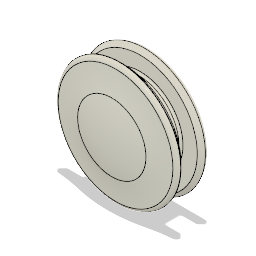
StepperBeltDisc v8 (Autodesk Fusion 360 design; units mm, degrees)
Autodesk Fusion 360 part; units mm, degrees
note: some values were not read from the file. Chosen so that the rebuilt part matches the saved one: which face or edge a step refers to; which pieces of a blend or face edit are solid. Set by a fixed rule: which sketch regions a step uses.
sketch "Sketch1" plane through (0, 0, 0) normal (0, 0, 1) x (1, 0, 0)
  circle A0 centre (0, 0) radius 15
  dimension "d1" = 30
  constraint coincident A0.centre origin
  measures "d1" diameter of A0
extrude "Extrude1" add sketch "Sketch1" along normal blind 8
sketch "Sketch2" plane through (0, 0, 0) normal (1, 0, 0) x (0, 0, -1)
  line L0 (0, 15) -> (0, -15)
  line L1 (-2, 15) -> (-2, 10)
  line L2 (-2, 10) -> (-6, 10)
  line L3 (-6, 10) -> (-6, 15)
  line L4 (-6, 15) -> (-2, 15)
  dimension "d4" = 5
  constraint parallel L0 L1
  constraint perpendicular L1 L2
  constraint perpendicular L2 L3
  constraint perpendicular L1 L4
  measures "d4" distance of L1.start L1.end
revolve "Revolve1" cut sketch "Sketch2" angle 360 about axis through (0, 0, 1.75) along (0, 0, 1)
sketch "Sketch3" plane through (0, 0, 8) normal (0, 0, 1) x (1, 0, 0)
  circle A0 centre (0, 0) radius 15
  circle A1 centre (0, 0) radius 2.6
  line L0 (2.6, 0) -> (2.15, 0) construction
  line L1 (2.15, 1.462) -> (2.15, -1.462)
  dimension "d6" = 5.2
  dimension "d7" = 0.45
  constraint coincident A0.centre A1.centre
  constraint coincident A1 L0.start
  constraint horizontal L0
  constraint coincident A1 L1.start
  constraint coincident A1 L1.end
  constraint perpendicular L0 L1
  measures "d6" diameter of A1
  measures "d7" distance of L0.start L0.end
extrude "Extrude2" cut sketch "Sketch3" against normal blind 8 contours A1 L1 picked at (-0.7322, 0.1665)
sketch "Sketch4" plane through (0, 0, 8) normal (0, 0, 1) x (1, 0, 0)
  line L0 (2.15, 1.462) -> (2.15, -1.462)
  arc A0 (2.15, 1.462) -> (2.15, -1.462) centre (0, 0) ccw
  circle A1 centre (0, 0) radius 15
  circle A2 centre (0, 0) radius 5
  constraint concentric A0 A2
extrude "Extrude3" add sketch "Sketch4" along normal blind 2 contours L0 A0 | A2
fillet "Fillet1" radius 34.888 2 edges at (-4.6616, 1.8081, 8) (-4.6616, -1.8081, 10)
fillet "Fillet2" radius 0.5 2 edges at (-9.3233, 3.6162, 6) (-9.3233, 3.6162, 2)
fillet "Fillet3" radius 1 2 edges at (-13.9849, -5.4242, 8) (-13.9849, -5.4242, 0)
chamfer "Chamfer1" distance 1 angle 45 2 edges at (-13.9849, -5.4242, 6) (-13.9849, 5.4242, 2)
chamfer "Chamfer2" distance 0.5 angle 45 2 edges at (-2.6, 0, 0) (2.15, 0, 0)
fillet "Fillet4" radius 0.5 1 faces at (-0.7322, 0.1665, 8)
equation "d1 = 25 mm + 5 mm"
equation "d6 = 5 mm + 0.2 mm"
equation "d7 = 0.6 mm - 0.15 mm"
